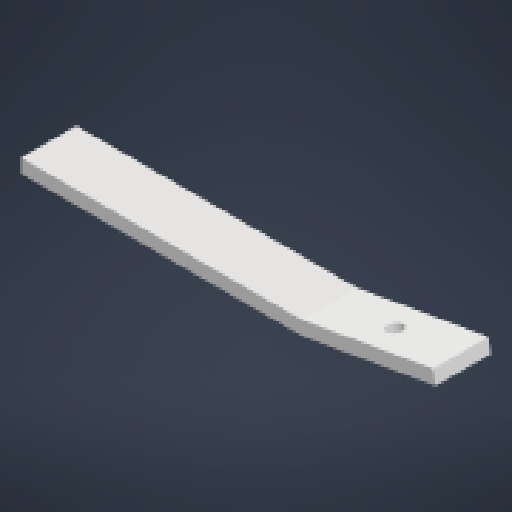
# Autodesk Inventor part: base mount for central centrifuge
Saved by Autodesk Inventor 2026 (Build 300175050, 175E)
## iProperties
Created: 2026-03-26
Part Number: base mount for central centrifuge
Material: Generic
Document SubType Name: Modeling
Designer: sniel
Density: 1 g/cm^3
Appearance: Default
Author: sniel
Autodesk Inventor part; units mm, degrees
ref_plane "YZ Plane" through (0, 0, 0) normal (1, 0, 0) x (0, 1, 0)
ref_plane "XZ Plane" through (0, 0, 0) normal (0, 1, 0) x (-1, 0, 0)
ref_plane "XY Plane" through (0, 0, 0) normal (0, 0, 1) x (1, 0, 0)
sketch "Sketch1" plane through (0, 0, 0) normal (0, 0, 1) x (1, 0, 0)
  line L0 (0, 0) -> (-50, 0)
  line L1 (-50, 0) -> (-50, -5)
  line L2 (-50, -5) -> (0, -5)
  line L3 (0, -5) -> (0, 0)
  line L4 (0, 0) -> (19.6962, 3.473)
  line L5 (0, 0) -> (20, 0) construction
  line L6 (19.6962, 3.473) -> (18.8279, 8.397)
  line L7 (18.8279, 8.397) -> (-28.7939, 0)
  line L8 (0, 0) -> (-28.3564, -5)
  line L9 (0, 0) -> (28.7939, 0) construction
  line L10 (-50, 0) -> (-130, 0)
  line L11 (-130, 0) -> (-130, -5)
  line L12 (-130, -5) -> (-50, -5)
  line L13 (18.8279, 8.397) -> (31, -5)
  line L14 (31, -5) -> (21, -5)
  line L15 (21, -5) -> (10.5825, 6.4659)
  line L16 (31, -5) -> (31, 0)
  line L17 (31, 0) -> (26.4572, 0)
  line L18 (31, 0) -> (36, 0)
  line L19 (36, 0) -> (36, -5)
  line L20 (36, -5) -> (31, -5)
  line L21 (31, -5) -> (31, 0)
  point P0 (14.1847, 2.5011)
  point P1 (31, -5)
  dimension "d0" = 50
  dimension "d1" = 5
  dimension "d2" = 20
  dimension "d3" = 10
  dimension "d4" = 5
  dimension "d5" = 90
  dimension "d11" = 170
  dimension "d12" = 80
  dimension "d16" = 5
  constraints: 44 end point, 6 horizontal, 6 perpendicular, 4 point on line, 3 parallel, 2 equal length, 2 vertical
  measures "d0" distance of L0.start L0.end
  measures "d1" distance of L0.end L1.end
  measures "d2" distance of L0.start L4.end
  measures "d3" angle of L5 L4
  measures "d4" distance of L4.end L6.end
  measures "d5" angle of L7 L6
  measures "d11" angle of L8 L9
  measures "d12" distance of L0.end L10.end
  measures "d16" distance of L13.end L16.end
extrude "Extrusion1" add sketch "Sketch1" along normal blind 20 contours L8 L2 L1 L0 | L0 L7 L6 L4 | L4 L6 L13 L14 L15 | L1 L12 L11 L10 | L17 L16 L13 | L16 L18 L19 L20
sketch "Sketch2" plane through (-28.7939, 0, 0) normal (-0.1736, 0.9848, 0) x (-0.9848, -0.1736, 0)
  line L0 (-48.3564, 0) -> (0, 0) projected
  line L1 (0, 0) -> (0, 20) projected
  line L2 (-48.3564, 20) -> (0, 20) projected
  line L3 (-48.3564, 0) -> (-48.3564, 20) projected
  line L4 (-48.3564, 10) -> (0, 10)
  line L5 (-24.1782, 20) -> (-24.1782, 0)
  line L6 (-28.3564, 0) -> (-48.3564, 0) projected
  circle A0 centre (-24.1782, 10) radius 2.75
  dimension "d8" = 5.5
  constraints: 4 end point, 4 midpoint, 1 centre point, 1 perpendicular, 1 point on line
  measures "d8" diameter of A0
extrude "Extrusion2" cut sketch "Sketch2" against normal blind 20 contours A0 L5 L4 | L4 L5 A0 | L5 L4 A0 | L5 A0 L4
sketch "Sketch3" plane through (0, 0, 0) normal (0, 1, 0) x (-1, 0, 0)
  line L0 (130, 0) -> (28.3564, 0) projected
  line L1 (28.3564, 0) -> (28.3564, 20) projected
  line L2 (130, 20) -> (28.3564, 20) projected
  line L3 (130, 0) -> (130, 20) projected
  line L4 (-18.8279, 0) -> (28.7939, 0) projected
  line L5 (28.3564, 20) -> (28.7939, 0)
  line L6 (28.3564, 0) -> (28.3564, 20) projected
  line L7 (28.3564, 10) -> (-19.6962, 10)
  line L8 (-19.6962, 0) -> (-19.6962, 20) projected
  line L9 (28.7939, 0) -> (130, 0) projected
  circle A0 centre (0, 10) radius 30.4809
  circle A1 centre (0, 10) radius 40
  point P0 (0, 0)
  point P1 (38.7298, 20)
  point P2 (38.7298, 0)
  point P3 (28.7939, 20)
  dimension "d13" = 80
  constraints: 4 end point, 2 midpoint, 1 centre point, 1 coincident, 1 point on line, 3 other
  measures "d13" diameter of A1
extrude "Extrusion3" add sketch "Sketch3" against normal blind 5 contours L0 A1 L2 A0 picked at (-11.3499, -24.8055)
body "Solid1"
